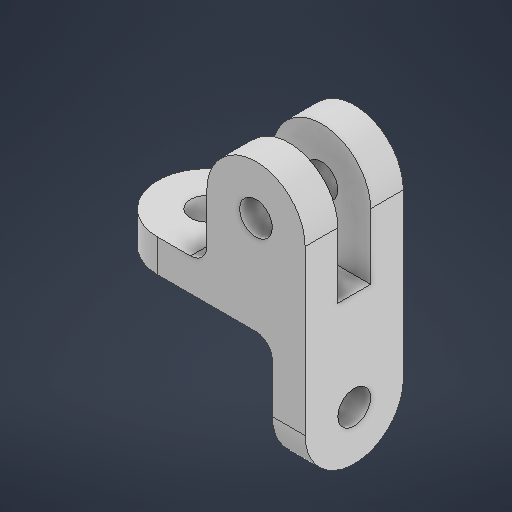
# Autodesk Inventor part: b5
Saved by Autodesk Inventor 2025.4 (Build 294407000, 407)
## iProperties
Created: 2026-05-07
Part Number: b5
Material: Generic
Document SubType Name: Modeling
Designer: VuQuan
Density: 1 g/cm^3
Appearance: Default
Author: VuQuan
Autodesk Inventor part; units mm, degrees
ref_plane "YZ Plane" through (0, 0, 0) normal (1, 0, 0) x (0, 1, 0)
ref_plane "XZ Plane" through (0, 0, 0) normal (0, 1, 0) x (-1, 0, 0)
ref_plane "XY Plane" through (0, 0, 0) normal (0, 0, 1) x (1, 0, 0)
sketch "Sketch1" plane through (0, 0, 0) normal (0, 0, 1) x (1, 0, 0)
  line L0 (0, 0) -> (45, 0)
  line L1 (50, -5) -> (50, -35)
  line L2 (50, -35) -> (60, -35)
  line L3 (60, -35) -> (60, 30)
  arc A0 (60, 30) -> (30, 30) centre (45, 30) ccw
  line L4 (30, 30) -> (30, 15.6159)
  line L5 (30, 15.6159) -> (30, 15)
  arc A1 (25, 10) -> (30, 15) centre (25, 15) ccw
  line L6 (25, 10) -> (0, 10)
  line L7 (0, 10) -> (0, 0)
  arc A2 (50, -5) -> (45, 0) centre (45, -5) ccw
  circle A3 centre (45, 30) radius 5
  dimension "d0" = 5
  dimension "d1" = 10
  dimension "d2" = 30
  dimension "d3" = 10
  dimension "d4" = 10
  dimension "d5" = 60
  dimension "d6" = 35
  dimension "d7" = 65
  constraints: 16 end point, 6 point on circle, 6 tangent, 5 perpendicular, 4 centre point, 2 coincident, 1 equal radius, 1 horizontal, 1 parallel, 1 point on line
  measures "d0" radius of A2
  measures "d1" distance of L1.end L2.end
  measures "d2" distance between parallel lines of L3 L4
  measures "d3" distance of L6.end L0.start
  measures "d4" diameter of A3
  measures "d5" distance between parallel lines of L3 L7
  measures "d6" distance between parallel lines of L0 L2
  measures "d7" distance from line of A0.centre L2
extrude "Extrusion1" add sketch "Sketch1" along normal blind 30
fillet "Fillet1" radius 15 4 edges at (0, 5, 30) (0, 5, 0) (55, -35, 30) (55, -35, 0)
sketch "Sketch2" plane through (60, 30, 30) normal (1, 0, 0) x (0, 0, -1)
  arc A0 (0, -50) -> (30, -50) centre (15, -50) ccw projected
  circle A1 centre (15, -50) radius 5
  line L0 (20, 15) -> (20, -20)
  line L1 (20, -20) -> (10, -20)
  line L2 (10, -20) -> (10, 15)
  line L3 (30, 15) -> (0, 15) projected
  line L4 (30, 15) -> (30, 0) projected
  line L5 (30, -20) -> (0, -20) projected
  point P0 (30, -30)
  point P1 (15, -20)
  point P2 (15, 15)
  point P3 (20, 15)
  dimension "d11" = 10
  dimension "d12" = 10
  constraints: 6 end point, 2 midpoint, 2 perpendicular, 1 centre point, 1 coincident, 1 collinear, 1 point on line, 1 vertical, 1 vertical alignment
  measures "d11" diameter of A1
  measures "d12" distance between parallel lines of L0 L4
extrude "Extrusion2" cut sketch "Sketch2" against normal through all
sketch "Sketch3" plane through (15, 10, 0) normal (0, 1, 0) x (1, 0, 0)
  arc A0 (0, 0) -> (0, -30) centre (0, -15) ccw projected
  circle A1 centre (0, -15) radius 5
  point P0 (-15, 0)
  dimension "d15" = 10
  constraints: 1 centre point, 1 coincident
  measures "d15" diameter of A1
extrude "Extrusion3" cut sketch "Sketch3" against normal through all
body "Solid1"
